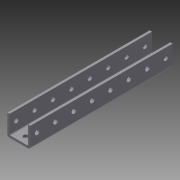
# Autodesk Inventor part: 8 in bar
Saved by Autodesk Inventor 2014 (Build 180170000, 170)
## iProperties
Created: 2014-01-06
Part Number: 8 in bar
Material: Generic
Document SubType Name: Modeling
Designer: Tristan Debrunner
Density: 1 g/cm^3
Appearance: Default
Author: Tristan Debrunner
Autodesk Inventor part; units mm, degrees
ref_plane "YZ Plane" through (0, 0, 0) normal (1, 0, 0) x (0, 1, 0)
ref_plane "XZ Plane" through (0, 0, 0) normal (0, 1, 0) x (-1, 0, 0)
ref_plane "XY Plane" through (0, 0, 0) normal (0, 0, 1) x (1, 0, 0)
sketch "Sketch1" plane through (0, 0, 0) normal (0, 0, 1) x (1, 0, 0)
  line L0 (3.175, 0) -> (28.575, 0)
  line L1 (31.75, 3.175) -> (31.75, 28.575)
  line L2 (0, 28.575) -> (0, 3.175)
  line L3 (4.7625, 3.175) -> (26.9875, 3.175)
  line L4 (28.575, 4.7625) -> (28.575, 28.575)
  line L5 (3.175, 28.575) -> (3.175, 4.7625)
  line L6 (0, 28.575) -> (3.175, 28.575)
  line L7 (28.575, 28.575) -> (31.75, 28.575)
  arc A0 (3.175, 4.7625) -> (4.7625, 3.175) centre (4.7625, 4.7625) ccw
  arc A1 (26.9875, 3.175) -> (28.575, 4.7625) centre (26.9875, 4.7625) ccw
  arc A2 (0, 3.175) -> (3.175, 0) centre (3.175, 3.175) ccw
  arc A3 (28.575, 0) -> (31.75, 3.175) centre (28.575, 3.175) ccw
  point P0 (0, 0)
  point P1 (0, 0)
  point P2 (31.75, 0)
  dimension "d0" = 31.75
  dimension "d1" = 28.575
  dimension "d2" = 1.5875
  dimension "d3" = 3.175
  constraints: 16 end point, 8 point on circle, 8 tangent, 4 centre point, 4 perpendicular, 4 point on line, 2 equal radius, 2 parallel, 1 horizontal
  measures "d0" distance of L2.start L7.end
  measures "d1" distance of L7.end point (31.75, 0)
  measures "d2" radius of A0
  measures "d3" radius of A2
extrude "Extrusion1" add sketch "Sketch1" along normal blind 196.85
sketch "Sketch2" plane through (31.75, 3.175, 0) normal (1, 0, 0) x (0, 0, -1)
  line L0 (-196.85, 0) -> (-196.85, 25.4) projected
  line L1 (0, 0) -> (-196.85, 0) projected
  line L2 (-196.85, 12.7) -> (-187.325, 12.7)
  point P0 (0, -3.175)
  dimension "d6" = 9.525
  constraints: 2 end point, 1 midpoint, 1 parallel
  measures "d6" distance of L2.start L2.end
sketch "Sketch3" plane through (3.175, 0, 0) normal (0, -1, 0) x (1, 0, 0)
  line L0 (0, 196.85) -> (25.4, 196.85) projected
  line L1 (0, 0) -> (0, 196.85) projected
  line L2 (12.7, 196.85) -> (12.7, 187.325)
  point P0 (-3.175, 0)
  dimension "d7" = 9.525
  constraints: 2 end point, 1 midpoint, 1 parallel
  measures "d7" distance of L2.start L2.end
hole "Hole1" at (31.75, 15.875, 187.325) direction (-1, 0, 0) diameter 6.35 end through all
hole "Hole2" at (15.875, 0, 187.325) direction (0, 1, 0) diameter 6.35 end through all
pattern_linear "Rectangular Pattern1" count 8 spacing 25.4 along (0, 0, -1) of "Hole1", "Hole2"
body "Solid1"
